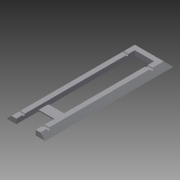
# Autodesk Inventor part: LegHolderV4
Saved by Autodesk Inventor 2014 (Build 180170000, 170)
## iProperties
Created: 2014-04-26
Part Number: LegHolderV4
Material: Generic
Document SubType Name: Modeling
Designer: Max
Density: 1 g/cm^3
Appearance: Default
Author: Max
Autodesk Inventor part; units mm, degrees
ref_plane "YZ Plane" through (0, 0, 0) normal (1, 0, 0) x (0, 1, 0)
ref_plane "XZ Plane" through (0, 0, 0) normal (0, 1, 0) x (-1, 0, 0)
ref_plane "XY Plane" through (0, 0, 0) normal (0, 0, 1) x (1, 0, 0)
sketch "Sketch1" plane through (0, 0, 0) normal (0, 1, 0) x (-1, 0, 0)
  line L0 (19.05, 63.5) -> (19.05, -63.5)
  line L1 (19.05, -63.5) -> (-19.05, -63.5)
  line L2 (-19.05, -63.5) -> (-19.05, 63.5)
  line L3 (9.525, 63.5) -> (9.525, -53.975)
  line L4 (9.525, -53.975) -> (-9.525, -53.975)
  line L5 (-9.525, -53.975) -> (-9.525, 63.5)
  line L6 (-19.05, 63.5) -> (-9.525, 63.5)
  line L7 (9.525, 63.5) -> (19.05, 63.5)
  line L8 (-9.525, 41.275) -> (9.525, 41.275)
  line L9 (9.525, 41.275) -> (9.525, 31.75)
  line L10 (9.525, 31.75) -> (-9.525, 31.75)
  line L11 (-9.525, 31.75) -> (-9.525, 41.275)
  point P0 (0, 0)
  dimension "d0" = 38.1
  dimension "d3" = 63.5
  dimension "d4" = 19.05
  dimension "d7" = 9.525
  dimension "d8" = 9.525
  dimension "d10" = 9.525
  dimension "d11" = 127
  dimension "d17" = 9.525
  dimension "d18" = 31.75
  constraints: 24 end point, 6 parallel, 3 horizontal, 3 perpendicular, 2 point on line, 1 collinear
  measures "d0" distance between parallel lines of L0 L2
  measures "d3" distance from line of L1 point (0, 0)
  measures "d4" distance from line of L2 point (0, 0)
  measures "d7" distance between parallel lines of L2 L5
  measures "d8" distance between parallel lines of L0 L3
  measures "d10" distance between parallel lines of L1 L4
  measures "d11" distance between parallel lines of L1 L7
  measures "d17" distance between parallel lines of L10 L8
  measures "d18" distance from line of point (0, 0) L10
extrude "Extrusion2" add sketch "Sketch1" along normal blind 4.7625 contours L0 L1 L2 L6 L5 L4 L3 L7
extrude "Extrusion3" add sketch "Sketch1" along normal blind 1.27 contours L3 L10 L5 L8
chamfer "Chamfer1" distance 4.7625 angle 45 3 edges at (19.05, 4.7625, 0) (-19.05, 4.7625, 0) (0, 4.7625, -63.5)
sketch "Sketch2" plane through (0, 0, 0) normal (1, 0, 0) x (0, 1, 0)
  line L0 (0, -63.5) -> (0, -53.975) projected
  line L1 (0, -53.975) -> (4.7625, -53.975) projected
  line L2 (1.27, 31.75) -> (0, 31.75) projected
  line L3 (0, 31.75) -> (0, 41.275) projected
  line L4 (0, 41.275) -> (1.27, 41.275) projected
  line L5 (1.27, 41.275) -> (1.27, 31.75) projected
  line L6 (1.27, 31.75) -> (0, 31.75) projected
  line L7 (0, 31.75) -> (0, -53.975) projected
  line L8 (0, -53.975) -> (4.7625, -53.975) projected
  line L9 (0, 63.5) -> (4.7625, 63.5) projected
  line L10 (0, 63.5) -> (0, 41.275) projected
  line L11 (0, 41.275) -> (1.27, 41.275) projected
  line L12 (1.27, 41.275) -> (1.27, 31.75) projected
  circle A0 centre (4.7625, 56.1022) radius 1.27
  circle A1 centre (4.7625, -46.3233) radius 1.27
  line L13 (4.7625, -53.975) -> (4.7625, -58.7375) projected
  line L14 (4.7625, -58.7375) -> (0, -63.5) projected
  line L15 (4.7625, 63.5) -> (4.7625, -53.975) projected
  point P0 (0, 0)
  point P1 (6.35, -57.15)
  point P2 (6.35, -57.15)
  dimension "d24" = 7.3978
  dimension "d25" = 7.6517
  dimension "d26" = 2.54
  dimension "d27" = 4.7625
  dimension "d28" = 4.7625
  constraints: 2 centre point, 1 equal radius, 1 other
  measures "d24" distance from line of L9 A0.centre
  measures "d25" distance from line of L1 A1.centre
  measures "d26" diameter of A0
  measures "d27" distance from line of L10 A0.centre
  measures "d28" distance from line of L7 A1.centre
extrude "Extrusion4" cut sketch "Sketch2" along normal through all both and the other way through all contours L15 A1 | A1 L15 | L15 A0 | A0 L15
equation "\"d3\" = 0.5 * d11"
equation "\"d4\" = 0.5 * d0"
equation "\"d8\" = d7"
equation "\"d10\" = d7"
equation "\"d17\" = d7"
equation "\"d18\" = 0.5 * d3"
equation "\"d12\" = 0.5 * d7"
equation "\"d14\" = 0.5 * d7"
equation "\"d27\" = 0.5 * d7"
equation "\"d28\" = d27"
equation "\"d22\" = 0.75 * d7"
body "Solid2"
